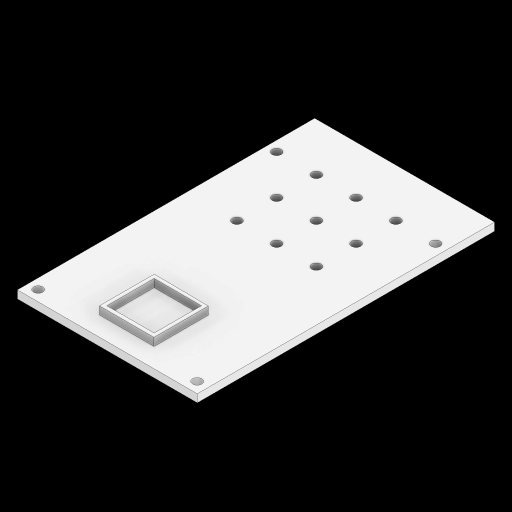
# Autodesk Inventor part: mounting_board_printed
Saved by Autodesk Inventor 2023 (Build 270158000, 158)
## iProperties
Created: 2024-07-03
Part Number: mounting_board_printed
Material: 일반
Document SubType Name: Modeling
Designer: OMS55
Density: 1 g/cm^3
Appearance: 기본값
Author: OMS55
Autodesk Inventor part; units mm, degrees
ref_plane "YZ Plane" through (0, 0, 0) normal (1, 0, 0) x (0, 1, 0)
ref_plane "XZ Plane" through (0, 0, 0) normal (0, 1, 0) x (-1, 0, 0)
ref_plane "XY Plane" through (0, 0, 0) normal (0, 0, 1) x (1, 0, 0)
sketch "스케치1" plane through (0, 0, 0) normal (0, 1, 0) x (-1, 0, 0)
  line L0 (0, 0) -> (-115, 0)
  line L1 (-115, 0) -> (-115, -190)
  line L2 (-115, -190) -> (0, -190)
  line L3 (0, -190) -> (0, 0)
  circle A0 centre (-6.5, -6.8) radius 2.95
  line L4 (0, -95) -> (-115, -95) construction
  line L5 (-57.5, 0) -> (-57.5, -190) construction
  circle A1 centre (-6.5, -183.2) radius 2.95
  circle A2 centre (-6.5, -32.2) radius 2.95
  circle A3 centre (-6.5, -57.6) radius 2.95
  circle A4 centre (-6.5, -83) radius 2.95
  circle A5 centre (-6.5, -108.4) radius 2.95
  circle A6 centre (-6.5, -133.8) radius 2.95
  circle A7 centre (-6.5, -159.2) radius 2.95
  circle A8 centre (-31.9, -6.8) radius 2.95
  circle A9 centre (-31.9, -32.2) radius 2.95
  circle A10 centre (-31.9, -57.6) radius 2.95
  circle A11 centre (-31.9, -83) radius 2.95
  circle A12 centre (-31.9, -108.4) radius 2.95
  circle A13 centre (-31.9, -133.8) radius 2.95
  circle A14 centre (-31.9, -159.2) radius 2.95
  circle A15 centre (-57.3, -6.8) radius 2.95
  circle A16 centre (-57.3, -32.2) radius 2.95
  circle A17 centre (-57.3, -57.6) radius 2.95
  circle A18 centre (-57.3, -83) radius 2.95
  circle A19 centre (-57.3, -108.4) radius 2.95
  circle A20 centre (-57.3, -133.8) radius 2.95
  circle A21 centre (-57.3, -159.2) radius 2.95
  circle A22 centre (-82.7, -6.8) radius 2.95
  circle A23 centre (-82.7, -32.2) radius 2.95
  circle A24 centre (-82.7, -57.6) radius 2.95
  circle A25 centre (-82.7, -83) radius 2.95
  circle A26 centre (-82.7, -108.4) radius 2.95
  circle A27 centre (-82.7, -133.8) radius 2.95
  circle A28 centre (-82.7, -159.2) radius 2.95
  circle A29 centre (-108.1, -6.8) radius 2.95
  circle A30 centre (-108.1, -32.2) radius 2.95
  circle A31 centre (-108.1, -57.6) radius 2.95
  circle A32 centre (-108.1, -83) radius 2.95
  circle A33 centre (-108.1, -108.4) radius 2.95
  circle A34 centre (-108.1, -133.8) radius 2.95
  circle A35 centre (-108.1, -159.2) radius 2.95
  circle A36 centre (-133.5, -6.8) radius 2.95
  circle A37 centre (-133.5, -32.2) radius 2.95
  circle A38 centre (-133.5, -57.6) radius 2.95
  circle A39 centre (-133.5, -83) radius 2.95
  circle A40 centre (-133.5, -108.4) radius 2.95
  circle A41 centre (-133.5, -133.8) radius 2.95
  circle A42 centre (-133.5, -159.2) radius 2.95
  dimension "d0" = 190
  dimension "d1" = 115
  dimension "d2" = 6.5
  dimension "d3" = 6.8
  dimension "d4" = 5.9
  dimension "d9" = 25.4
  dimension "d12" = 25.4
  constraints: 43 centre point, 12 end point, 4 midpoint, 2 horizontal, 2 parallel, 1 coincident, 1 perpendicular, 1 symmetric about line, 1 vertical, 83 other
  measures "d0" distance of L2.end L0.start
  measures "d1" distance of L1.end L2.end
  measures "d2" distance from line of L3 A0.centre
  measures "d3" distance from line of L0 A0.centre
  measures "d4" diameter of A0
  measures "d9" distance of A0.centre A2.centre
  measures "d12" distance of A0.centre A8.centre
extrude "돌출1" add sketch "스케치1" along normal blind 5 contours L3 L2 L1 L0 | A1 | A2 | A3 | A4 | A5 | A6 | A7 | A8 | A9 | A10 | A11 | A12 | A13 | A14 | A15 | A16 | A17 | A18 | A19 | A20 | A21 | A22 | A23 | A24 | A25 | A26 | A27 | A28 | A29 | A30 | A31 | A32 | A33 | A34 | A35
extrude "돌출2" cut sketch "스케치1" along normal blind 5 contours A12 | A13 | A14 | A19 | A20 | A21 | A26 | A27 | A28
extrude "돌출4" cut sketch "스케치1" along normal blind 5 contours A35
extrude "돌출5" cut sketch "스케치1" along normal blind 5 contours A7
sketch "스케치2" plane through (0, 5, 0) normal (0, 1, 0) x (1, 0, 0)
  circle A0 centre (57.5, 63.8) radius 2.5
  line L0 (0, 0) -> (115, 0) projected
  circle A1 centre (57.3, 133.8) radius 2.95 projected
  point P0 (57.5, 0)
  dimension "d23" = 70
  dimension "d24" = 5
  constraints: 1 centre point, 1 midpoint, 1 vertical alignment
  measures "d23" vertical distance of A1.centre A0.centre
  measures "d24" diameter of A0
extrude "돌출6" cut sketch "스케치1" along normal blind 5 contours A29
sketch "스케치3" plane through (0, 5, 0) normal (0, 1, 0) x (1, 0, 0)
  line L0 (42.4, 14.8) -> (72.6, 14.8)
  line L1 (72.6, 14.8) -> (72.6, 45)
  line L2 (72.6, 45) -> (42.4, 45)
  line L3 (42.4, 45) -> (42.4, 14.8)
  line L4 (115, 190) -> (0, 190) projected
  line L5 (40.0511, 12.35) -> (74.9489, 12.35)
  line L6 (74.9489, 12.35) -> (74.9489, 47.05)
  line L7 (74.9489, 47.05) -> (40.0511, 47.45)
  line L8 (40.0511, 47.45) -> (40.0511, 12.35)
  line L9 (0, 0) -> (115, 0) projected
  point P0 (57.5, 45)
  point P1 (57.5, 190)
  point P2 (57.5, 190)
  point P3 (57.5, 47.25)
  point P4 (57.5, 12.35)
  point P5 (40.0511, 29.9)
  point P6 (42.4, 29.9)
  dimension "d27" = 30.2
  dimension "d28" = 30.2
  dimension "d29" = 145
  dimension "d31" = 34.9
  dimension "d34" = 2.45
  dimension "d35" = 34.9
  constraints: 16 end point, 7 midpoint, 4 parallel, 2 vertical alignment, 1 horizontal, 1 horizontal alignment, 1 perpendicular
  measures "d27" distance of L2.end L0.start
  measures "d28" distance of L0.start L0.end
  measures "d29" distance of point (57.5, 190) point (57.5, 45)
  measures "d31" distance of L6.end L7.end
  measures "d34" distance between parallel lines of L0 L5
  measures "d35" distance of point (57.5, 47.25) point (57.5, 12.35)
extrude "돌출7" add sketch "스케치3" along normal blind 5
